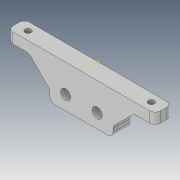
# Autodesk Inventor part: gripperPart3
Saved by Autodesk Inventor 2018 (Build 220112000, 112)
## iProperties
Created: 2020-01-19
Part Number: gripperPart3
Material: Generic
Document SubType Name: Modeling
Designer: anirudh
Density: 1 g/cm^3
Appearance: Default
Author: anirudh
Autodesk Inventor part; units mm, degrees
ref_plane "YZ Plane" through (0, 0, 0) normal (1, 0, 0) x (0, 1, 0)
ref_plane "XZ Plane" through (0, 0, 0) normal (0, 1, 0) x (-1, 0, 0)
ref_plane "XY Plane" through (0, 0, 0) normal (0, 0, 1) x (1, 0, 0)
sketch "Sketch1" plane through (0, 0, 0) normal (0, 0, 1) x (1, 0, 0)
  line L0 (0, 0) -> (88.9, 0)
  line L1 (44.45, -15.24) -> (25.4, -15.24)
  line L2 (25.4, -15.24) -> (63.5, -15.24)
  line L3 (0, 0) -> (0, -6.35)
  line L4 (0, -6.35) -> (25.4, -6.35)
  line L5 (25.4, -6.35) -> (25.4, -15.24)
  line L6 (63.5, -15.24) -> (63.5, -6.35)
  line L7 (63.5, -6.35) -> (88.9, -6.35)
  line L8 (88.9, -6.35) -> (88.9, 0)
  dimension "d0" = 88.9
  dimension "d3" = 19.05
  dimension "d4" = 38.1
  dimension "d5" = 6.35
  constraints: 18 end point, 3 perpendicular, 3 point on line, 2 horizontal, 1 parallel, 1 vertical
  measures "d0" distance of L0.start L0.end
  measures "d3" distance of L1.start L1.end
  measures "d4" distance of L1.end L2.end
  measures "d5" distance of L0.start L3.end
extrude "Extrusion1" add sketch "Sketch1" along normal blind 10
ref_plane "Work Plane1" through (44.45, -6.35, 0) normal (1, 0, 0) x (0, 0, -1)
sketch "Sketch2" plane through (0, 0, 10) normal (0, 0, 1) x (1, 0, 0)
  line L0 (25.4, -15.24) -> (63.5, -15.24) projected
  line L1 (25.4, -15.24) -> (63.5, -15.24)
  line L2 (63.5, -15.24) -> (63.5, -25.4)
  line L3 (63.5, -25.4) -> (25.4, -25.4)
  line L4 (25.4, -25.4) -> (25.4, -15.24)
  point P0 (0, 0)
  dimension "d8" = 10.16
  constraints: 8 end point, 2 parallel, 1 horizontal, 1 perpendicular
  measures "d8" distance of L1.end L2.end
extrude "Extrusion2" add sketch "Sketch2" against normal blind 10
sketch "Sketch3" plane through (0, 0, 10) normal (0, 0, 1) x (1, 0, 0)
  line L0 (63.5, -25.4) -> (25.4, -25.4) projected
  line L1 (25.4, -25.4) -> (63.5, -25.4)
  line L2 (63.5, -25.4) -> (25.4, -25.4) projected
  line L3 (25.4, -25.4) -> (44.45, -25.4)
  line L4 (44.45, -25.4) -> (63.5, -25.4)
  circle A0 centre (34.925, -16.86) radius 3.05
  circle A1 centre (53.975, -16.86) radius 3.05
  point P0 (0, 0)
  dimension "d31" = 6.1
  dimension "d32" = 6.1
  constraints: 6 end point, 2 centre point, 2 collinear, 1 midpoint
  measures "d31" diameter of A0
  measures "d32" diameter of A1
extrude "Extrusion3" cut sketch "Sketch3" against normal blind 25.4
chamfer "Chamfer1" distance 12.7 angle 45 2 edges at (25.4, -6.35, 5) (63.5, -6.35, 5)
fillet "Fillet1" radius 3.175 10 edges at (0, -3.175, 0) (0, -3.175, 10) (12.7, -6.35, 5) (25.4, -19.05, 5) (25.4, -25.4, 5) (63.5, -25.4, 5) (63.5, -19.05, 5) (76.2, -6.35, 5) (88.9, -3.175, 10) (88.9, -3.175, 0)
sketch "Sketch4" plane through (3.175, 0, 0) normal (0, 1, 0) x (1, 0, 0)
  circle A0 centre (78.4451, -5) radius 1.8
  circle A1 centre (4.1049, -5) radius 1.8
  point P0 (-3.175, 0)
  point P1 (8.2099, -10)
  point P2 (0, 0)
  point P3 (82.55, -10)
  point P4 (74.3401, 0)
  dimension "d27" = 3.6
  dimension "d28" = 3.6
  constraints: 2 centre point
  measures "d27" diameter of A0
  measures "d28" diameter of A1
extrude "Extrusion4" cut sketch "Sketch4" against normal blind 25.4
body "Solid1"
